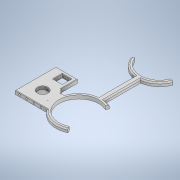
# Autodesk Inventor part: backplate with potentiometer
Saved by Autodesk Inventor 2022 (Build 260153000, 153)
## iProperties
Created: 2021-11-11
Part Number: backplate with potentiometer
Material: Generic
Document SubType Name: Modeling
Designer: a-dubs
Density: 1 g/cm^3
Appearance: Default
Author: a-dubs
Autodesk Inventor part; units mm, degrees
ref_plane "YZ Plane" through (0, 0, 0) normal (1, 0, 0) x (0, 1, 0)
ref_plane "XZ Plane" through (0, 0, 0) normal (0, 1, 0) x (-1, 0, 0)
ref_plane "XY Plane" through (0, 0, 0) normal (0, 0, 1) x (1, 0, 0)
sketch "Sketch1" plane through (0, 0, 0) normal (0, 1, 0) x (-1, 0, 0)
  circle A0 centre (0, 0) radius 32.5
  line L0 (0, 32.5) -> (0, 102.5)
  line L1 (0, 102.5) -> (0, 169.7)
  circle A1 centre (0, 136.1) radius 33.6
  circle A2 centre (0, 136.1) radius 42.65
  line L2 (42.65, 136.0981) -> (38.65, 136.0981)
  line L3 (38.65, 136.0981) -> (61.05, 136.0981)
  circle A3 centre (61.05, 136.0981) radius 22.4
  line L4 (61.05, 136.0981) -> (61.05, 134.1981)
  line L5 (61.05, 136.0981) -> (61.05, 137.9981)
  circle A4 centre (61.05, 136.0981) radius 2.8
  line L6 (61.05, 137.9981) -> (63.1067, 137.9981)
  line L7 (61.05, 137.9981) -> (58.9933, 137.9981)
  line L8 (61.05, 134.1981) -> (58.9933, 134.1981)
  line L9 (61.05, 134.1981) -> (63.1067, 134.1981)
  circle A5 centre (61.05, 136.0981) radius 4.7
  line L10 (0, -32.5) -> (0, -37.5)
  circle A6 centre (0, 0) radius 37.5
  line L11 (0, 32.5) -> (5, 32.5)
  line L12 (5, 32.5) -> (5, 93.7441)
  line L13 (0, 32.5) -> (-5, 32.5)
  line L14 (-5, 32.5) -> (-5, 93.7441)
  line L15 (0, 0) -> (29.257, 0) construction
  line L16 (0, 0) -> (37.5, 0) construction
  line L17 (0, 0) -> (35.2385, 12.8258)
  line L18 (0, 0) -> (37.5, 0) construction
  line L19 (0, 0) -> (-35.2385, 12.8258)
  line L20 (0, 0) -> (37.5, 0) construction
  line L21 (0, 169.7) -> (0, 174.7)
  circle A7 centre (0, 136.1) radius 38.6
  line L22 (5, 93.7441) -> (5, 102.8741)
  line L23 (-5, 93.7441) -> (-5, 102.8741)
  line L24 (0, 136.1) -> (-18.0247, 97.446)
  line L25 (0, 136.1) -> (42.65, 136.1) construction
  line L26 (0, 136.1) -> (-18.0247, 174.754)
  line L27 (0, 136.1) -> (42.65, 136.1) construction
  circle A8 centre (61.05, 136.0981) radius 8.2
  line L28 (61.0525, 127.8981) -> (61.0525, 124.8981)
  line L29 (69.25, 136.0981) -> (72.25, 136.0981)
  line L30 (61.05, 144.2981) -> (61.05, 147.2981)
  line L31 (61.05, 147.2981) -> (72.25, 147.2981)
  line L32 (72.25, 147.2981) -> (72.25, 136.0981)
  line L33 (72.25, 124.8981) -> (72.25, 136.0981)
  line L34 (61.0525, 124.8981) -> (72.25, 124.8981)
  line L35 (61.0525, 124.8981) -> (31.6777, 124.8981)
  line L36 (61.05, 147.2981) -> (31.6784, 147.3)
  line L37 (61.0525, 127.8981) -> (61.0525, 129.4981)
  line L38 (61.0525, 129.4981) -> (60.2525, 129.4981)
  line L39 (60.2525, 129.4981) -> (61.8525, 129.4981)
  line L40 (61.8525, 129.4981) -> (61.8525, 127.9375)
  line L41 (60.2525, 127.937) -> (60.2525, 129.4981)
  line L42 (52.85, 136.0981) -> (49.85, 136.0981)
  line L43 (49.85, 136.0981) -> (49.85, 124.8981)
  line L44 (49.85, 147.2989) -> (49.85, 136.0981)
  line L45 (61.0525, 124.8981) -> (68.5525, 124.8981)
  line L46 (61.05, 136.0981) -> (61.05, 110.5981)
  line L47 (61.05, 110.5981) -> (68.5525, 110.5981)
  line L48 (53.55, 110.5981) -> (61.05, 110.5981)
  line L49 (72.25, 124.8981) -> (72.25, 97.446)
  line L50 (72.25, 97.446) -> (49.85, 97.446)
  line L51 (49.85, 97.446) -> (49.85, 124.8981)
  line L52 (49.85, 97.446) -> (47.85, 97.446)
  line L53 (72.25, 97.446) -> (74.25, 97.446)
  line L54 (74.25, 97.446) -> (74.25, 95.446)
  line L55 (74.25, 95.446) -> (47.85, 95.446)
  line L56 (47.85, 95.446) -> (47.85, 118.0006)
  line L57 (47.85, 118.0006) -> (74.25, 118.0006)
  line L58 (74.25, 118.0006) -> (74.25, 95.446)
  line L59 (74.25, 118.0006) -> (72.25, 124.8981)
  line L60 (47.85, 118.0006) -> (49.85, 124.8981)
  line L61 (61.05, 110.5981) -> (61.05, 95.5981)
  line L62 (61.05, 95.5981) -> (61.05, 90.5981)
  line L63 (61.05, 90.5981) -> (47.85, 90.5981)
  line L64 (47.85, 90.5981) -> (47.85, 95.446)
  line L65 (74.25, 95.446) -> (74.25, 90.5981)
  line L66 (74.25, 90.5981) -> (61.05, 90.5981)
  line L67 (68.5525, 110.5981) -> (68.5525, 95.5981)
  line L68 (68.5525, 95.5981) -> (53.55, 95.5981)
  line L69 (53.55, 95.5981) -> (53.55, 110.5981)
  line L70 (72.25, 147.2981) -> (84.25, 147.2981)
  line L71 (84.25, 147.2981) -> (84.25, 90.5981)
  line L72 (84.25, 90.5981) -> (74.25, 90.5981)
  line L73 (84.25, 147.2981) -> (84.25, 159.2981)
  line L74 (84.25, 159.2981) -> (30.8514, 159.2981)
  line L75 (30.8514, 159.2981) -> (24.3065, 159.2981)
  point P0 (37.3613, 126.4)
  point P1 (41.3137, 146.6924)
  point P2 (41.3131, 125.5051)
  point P3 (5, 97.8252)
  point P4 (-5, 97.8252)
  point P5 (-16.3131, 171.0835)
  point P6 (-14.2, 166.5519)
  point P7 (-14.2, 105.6481)
  point P8 (-16.3131, 101.1165)
  point P9 (5, 37.1652)
  point P10 (36.9388, 124.8981)
  point P11 (41.1527, 124.8981)
  point P12 (41.651, 124.8981)
  point P13 (41.6517, 147.2994)
  point P14 (41.1533, 147.2994)
  point P15 (36.9395, 147.2997)
  point P16 (-5, 37.1652)
  point P17 (-30.54, 11.1157)
  point P18 (30.54, 11.1157)
  point P19 (49.85, 116.6992)
  point P20 (53.55, 97.446)
  point P21 (68.5525, 97.446)
  dimension "d0" = 65
  dimension "d1" = 70
  dimension "d2" = 67.2
  dimension "d3" = 85.3
  dimension "d4" = 4
  dimension "d6" = 22.4
  dimension "d7" = 1.9
  dimension "d8" = 1.9
  dimension "d9" = 5.6
  dimension "d10" = 9.4
  dimension "d11" = 5
  dimension "d12" = 5
  dimension "d13" = 5
  dimension "d16" = 20
  dimension "d17" = 160
  dimension "d18" = 5
  dimension "d28" = 115
  dimension "d29" = 115
  dimension "d30" = 16.4
  dimension "d31" = 3
  dimension "d32" = 3
  dimension "d33" = 3
  dimension "d34" = 1.6
  dimension "d35" = 0.8
  dimension "d36" = 1.6
  dimension "d39" = 3
  dimension "d54" = 7.5
  dimension "d56" = 25.5
  dimension "d67" = 2
  dimension "d68" = 2
  dimension "d69" = 2
  dimension "d73" = 15
  dimension "d74" = 5
  dimension "d75" = 12
  dimension "d76" = 12
  constraints: 152 end point, 30 point on circle, 18 horizontal, 16 perpendicular, 15 point on line, 15 vertical, 9 centre point, 8 coincident, 7 parallel, 4 collinear, 4 equal length, 2 midpoint, 1 tangent
  measures "d0" diameter of A0
  measures "d1" distance of L0.start L0.end
  measures "d2" distance of L0.end L1.end
  measures "d3" diameter of A2
  measures "d4" distance of L2.start L2.end
  measures "d6" distance of L2.end L3.end
  measures "d7" distance of L4.start L4.end
  measures "d8" distance of L4.start L5.end
  measures "d9" diameter of A4
  measures "d10" diameter of A5
  measures "d11" distance of L10.start L10.end
  measures "d12" distance of L0.start L11.end
  measures "d13" distance of L0.start L13.end
  measures "d16" angle of L18 L17
  measures "d17" angle of L20 L19
  measures "d18" distance of L1.end L21.end
  measures "d28" angle of L24 L25
  measures "d29" angle of L27 L26
  measures "d30" diameter of A8
  measures "d31" distance of L28.start L28.end
  measures "d32" distance of L29.start L29.end
  measures "d33" distance of L30.start L30.end
  measures "d34" distance of L28.start L37.end
  measures "d35" distance of L37.end L38.end
  measures "d36" distance of L38.end L39.end
  measures "d39" distance of L42.start L42.end
  measures "d54" distance of L28.end L45.end
  measures "d56" distance of L46.start L46.end
  measures "d67" distance of L50.end L52.end
  measures "d68" distance of L49.end L53.end
  measures "d69" distance of L53.end L54.end
  measures "d73" distance of L46.end L61.end
  measures "d74" distance of L61.end L62.end
  measures "d75" distance of L31.end L70.end
  measures "d76" distance of L70.end L73.end
extrude "Extrusion4" add sketch "Sketch1" along normal blind 6 contours L19 A6 L14 L13 A0 | A0 L11 L12 A6 L17 | L13 L14 A6 L0 | L0 A6 L12 L11 | A6 L14 A2 L0 | L0 A2 L12 A6 | A2 L23 A7 L0 | L0 A7 L22 A2 | A7 L23 A1 L0 | L0 A1 L22 A7 | A7 L24 A1 L23 | L35 A7 L36 A2 A3 | L22 A1 L35 A7 | A3 L2 A2 | A2 L3 L43 L35 A3 | L35 A1 L36 A7 | A7 L21 A1 L26 | L2 A3 A2 | A2 A3 L36 L44 L3 | L21 A7 L75 A1 | A7 L36 A1 L75
extrude "Extrusion5" cut sketch "Sketch1" along normal blind 1.5 contours A8 L40 L39 L38 L46 A5 L3 | L3 A5 L46 L38 L41 A8 | L46 L38 L37 A8 | A8 L41 L38 L46 | A5 L46 A4 L3 | L3 A4 L46 A5 | L37 L39 L40 A8 | A4 L7 L5 L3 | L3 L4 L8 A4 | L5 L6 A4 L9 L4 | A4 L6 L7 | L8 L46 A4 | L46 L9 A4
extrude "Extrusion6" add sketch "Sketch1" along normal blind 1.5 contours A8 L40 L39 L38 L46 A5 L3 | L3 A5 L46 L38 L41 A8 | L46 L38 L37 A8 | A8 L41 L38 L46 | A5 L46 A4 L3 | L3 A4 L46 A5 | L37 L39 L40 A8 | A4 L7 L5 L3 | L3 L4 L8 A4 | L5 L6 A4 L9 L4 | A4 L6 L7 | L8 L46 A4 | L46 L9 A4
extrude "Extrusion7" add sketch "Sketch1" along normal blind 1.6 from surface at 1.5 contours L46 L38 L37 A8 | A8 L41 L38 L46 | L37 L39 L40 A8
extrude "Extrusion8" add sketch "Sketch1" along normal blind 4.5 and the other way blind 1.5 from surface at 1.5 contours L43 L3 A8 L46 L35 | L44 L36 L30 A8 L3 | L46 A8 L28 L35 | L28 A8 L29 L33 L34 | L30 L31 L32 L29 A8
extrude "Extrusion9" add sketch "Sketch1" along normal blind 6 contours L35 L60 A3 | L57 L51 A3 | A3 L51 L52 L56 | L60 L51 L57 | L35 L46 L57 L51 | L51 L57 L46 A3 | A3 L46 L48 L69 L50 L51 | L52 L50 L69 L68 L62 L55 L56 | L35 L34 L49 L57 L46 | L46 L57 L49 A3 | A3 L49 L50 L67 L47 L46 | L55 L62 L63 L64 | L49 L57 A3 | A3 L58 L53 L49 | L62 L68 L67 L50 L53 L54 L55 | L55 L65 L66 L62 | L49 L59 L57
chamfer "Chamfer3" distance 2 angle 45 7 edges at (-24.959, 6, 106.655) (10.7829, 6, 99.0367) (-5, 6, 67.4952) (5, 6, 67.4952) (-15.741, 6, 171.3446) (-23.5135, 6, 29.2124) (23.5135, 6, 29.2124)
extrude "Extrusion10" add sketch "Sketch1" along normal blind 6 contours L74 L73 L70 A3 L36 A2 | A2 L36 A7 L74 | A7 L36 A1 L75 | A3 L70 L31 L36 | L71 L72 L65 L54 L58 A3 L70 | A3 L59 L33 L32 L70
sketch "Sketch2" plane through (-84.25, 0, 90.5981) normal (-1, 0, 0) x (0, 0, 1)
  line L0 (68.7, 0) -> (68.7, 6) projected
  line L1 (0, 0) -> (68.7, 0)
  line L2 (68.7, 0) -> (68.7, 6)
  line L3 (68.7, 6) -> (0, 6)
  line L4 (0, 6) -> (0, 0)
  line L5 (0, 0) -> (0, 6) projected
  line L6 (0, 3) -> (2.35, 3)
  line L7 (34.3, 0) -> (34.3, 6) projected
  line L8 (34.3, 6) -> (34.3, 0)
  line L9 (68.6, 3) -> (66.25, 3)
  line L10 (2.35, 3) -> (3.95, 3)
  circle A0 centre (3.95, 3) radius 1.6
  circle A1 centre (15.95, 3) radius 1.6
  circle A2 centre (27.95, 3) radius 1.6
  circle A3 centre (39.95, 3) radius 1.6
  circle A4 centre (51.95, 3) radius 1.6
  circle A5 centre (63.95, 3) radius 1.6
  point P0 (-90.5981, 0)
  dimension "d79" = 2.35
  dimension "d82" = 1.6
  dimension "d83" = 3.2
  dimension "d86" = 12
  constraints: 16 end point, 6 centre point, 4 perpendicular, 3 horizontal, 2 symmetric about line, 1 coincident, 1 collinear, 1 midpoint, 10 other
  measures "d79" distance of L6.start L6.end
  measures "d82" distance of L6.end L10.end
  measures "d83" diameter of A0
  measures "d86" distance of A0.centre A1.centre
extrude "Extrusion11" cut sketch "Sketch2" against normal blind 5 contours A0 | A1 | A2 | A3 | A4 | A5
sketch "Sketch3" plane through (-84.25, 0, 159.2981) normal (0, 0, 1) x (1, 0, 0)
  line L0 (0, 0) -> (0, 6) projected
  line L1 (0, 0) -> (0, 6)
  line L2 (0, 6) -> (0, 3)
  line L3 (0, 3) -> (6, 3)
  line L4 (6, 3) -> (7.6, 3)
  circle A0 centre (7.6, 3) radius 1.6
  circle A1 centre (19.6, 3) radius 1.6
  circle A2 centre (31.6, 3) radius 1.6
  circle A3 centre (43.6, 3) radius 1.6
  point P0 (84.25, 0)
  dimension "d93" = 6
  dimension "d94" = 1.6
  dimension "d95" = 3.2
  dimension "d98" = 12
  constraints: 8 end point, 4 centre point, 2 horizontal, 1 coincident, 1 collinear, 1 midpoint, 1 perpendicular, 6 other
  measures "d93" distance of L2.end L3.end
  measures "d94" distance of L3.end L4.end
  measures "d95" diameter of A0
  measures "d98" distance of A0.centre A1.centre
extrude "Extrusion12" cut sketch "Sketch3" against normal blind 5
sketch "Sketch4" plane through (-47.85, 0, 90.5981) normal (0, 0, -1) x (-1, 0, 0)
  line L0 (36.4, 0) -> (36.4, 6) projected
  line L1 (36.4, 0) -> (0.047, 0)
  line L2 (36.4, 0) -> (-16.9986, 0) projected
  line L3 (36.4, 6) -> (36.4, 0)
  line L4 (36.4, 0) -> (36.4, 6) projected
  line L5 (36.4, 3) -> (30.4, 3)
  circle A0 centre (28.8, 3) radius 1.6 projected
  line L6 (30.4, 3) -> (28.8, 3)
  circle A1 centre (28.8, 3) radius 1.6
  circle A2 centre (16.8, 3) radius 1.6
  circle A3 centre (4.8, 3) radius 1.6
  point P0 (-47.85, 0)
  dimension "d105" = 6
  dimension "d108" = 12
  constraints: 8 end point, 3 centre point, 3 horizontal, 1 coincident, 1 collinear, 1 horizontal alignment, 1 midpoint, 1 point on line, 5 other
  measures "d105" distance of L5.start L5.end
  measures "d108" distance of A1.centre A2.centre
extrude "Extrusion13" cut sketch "Sketch4" against normal blind 5
chamfer "Chamfer5" distance 0.75 angle 45 11 edges at (-66.05, 6, 90.5981) (-47.85, 6, 104.2994) (-84.25, 6, 124.9481) (-56.2796, 6, 159.2981) (-44.1595, 6, 121.3852) (-37.9981, 6, 124.8981) (-52.85, 6, 136.0981) (-61.0513, 6, 110.5981) (-53.55, 6, 103.0981) (-68.5525, 6, 103.0981) (-61.0513, 6, 95.5981)
body "Solid2"
